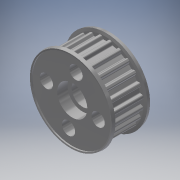
# Autodesk Inventor part: Synchrone Riemenscheibe2
Saved by Autodesk Inventor 2018.3 (Build 223284000, 284)
## iProperties
Created: 2018-08-12
Part Number: Synchrone Riemenscheibe2
Material: Steel
Document SubType Name: Modeling
Designer: JochenAlt
Density: 1 g/cm^3
Appearance: Steel
CustomPartVersion: 1
Author: JochenAlt
Autodesk Inventor part; units mm, degrees
ref_plane "YZ Plane" through (0, 0, 0) normal (1, 0, 0) x (0, 1, 0)
ref_plane "XZ Plane" through (0, 0, 0) normal (0, 1, 0) x (-1, 0, 0)
ref_plane "XY Plane" through (0, 0, 0) normal (0, 0, 1) x (1, 0, 0)
sketch "Riemenscheibenskizze" plane through (0, 0, 0) normal (0, 0, 1) x (1, 0, 0)
  circle A0 centre (0, 0) radius 9.5493 construction
  circle A1 centre (0, 0) radius 9.2493
  circle A2 centre (0, 0) radius 8.4993
  line L0 (-0.8562, 9.2096) -> (-0.525, 8.4993)
  line L1 (-0.525, 8.4993) -> (0.525, 8.4993)
  line L2 (0.525, 8.4993) -> (0.8562, 9.2096)
  line L3 (0, 0) -> (0, 9.2493) construction
  point P0 (0, 8.4993)
  dimension "d0" = 19.0986
  dimension "d1" = 0.3
  dimension "d2" = 0.75
  dimension "d3" = 50
  dimension "d4" = 1.05
  constraints: 8 end point, 3 coincident, 3 point on circle, 2 centre point, 1 horizontal, 1 midpoint, 1 point on line, 1 vertical, 1 vertical alignment, 3 other
  measures "d0" diameter of A0
  measures "d1" radial gap between concentric circles of A0 A1
  measures "d3" angle of L2 L0
  measures "d4" distance of L0.end L1.end
extrude "Grundkörper" add sketch "Riemenscheibenskizze" along normal mid plane 7.5 contours A2 | A1 L0 L1 L2 | L2 L1 L0 A1
extrude "Zahn" cut sketch "Riemenscheibenskizze" along normal through all both and the other way through all contours L2 L1 L0 A1 picked at (0, 8.9964)
fillet "Fillet" radius 0.2 2 edges at (0.525, 8.4993, 0) (-0.525, 8.4993, 0)
fillet "Fillet" radius 0.3 4 edges at (-0.8562, 9.2096, 1.875) (-0.8562, 9.2096, -1.875) (0.8562, 9.2096, 1.875) (0.8562, 9.2096, -1.875)
pattern_circular "Zähne" count 24 over 360 about axis through (0, 0, -10) along (0, 0, 1) of "Zahn", "Fillet"
pulley flange "Flansch links" diameter 18.4986 height 0.8 thickness 0.8 bend angle 10 centre (0, 0, -3.75) toward (0, 0, -1)
pulley flange "Flansch rechts" diameter 18.4986 height 0.8 thickness 0.8 bend angle 10 centre (0, 0, 3.75) toward (0, 0, 1)
sketch "Skizze3" plane through (0, 0, -4.55) normal (0, 0, -1) x (-1, 0, 0)
  circle A0 centre (0, 0) radius 6.35 construction
  line L0 (-14.069, 0) -> (14.069, 0) construction
  circle A1 centre (-0.9037, 6.2854) radius 1.6
  circle A2 centre (0, 0) radius 10.0493 projected
  circle A3 centre (0, 0) radius 9.6
  line L1 (0, -14.069) -> (0, 14.069) construction
  line L2 (14.069, 0) -> (-14.069, 0) construction
  line L3 (0, 0) -> (-0.9037, 6.2854) construction
  circle A4 centre (0, 0) radius 3.65
  circle A5 centre (0, 0) radius 2.65
  circle A6 centre (-0.9037, 6.2854) radius 2.5
  circle A7 centre (-6.2854, -0.9037) radius 1.6
  circle A8 centre (-6.2854, -0.9037) radius 2.5
  circle A9 centre (0.9037, -6.2854) radius 1.6
  circle A10 centre (0.9037, -6.2854) radius 2.5
  circle A11 centre (6.2854, 0.9037) radius 1.6
  circle A12 centre (6.2854, 0.9037) radius 2.5
  dimension "d24" = 6.35
  dimension "d25" = 3.2
  dimension "d30" = 19.2
  dimension "d35" = 8.182
  dimension "d36" = 7.3
  dimension "d38" = 1
  dimension "d43" = 5
  dimension "d46" = 360
  constraints: 12 centre point, 5 coincident, 2 end point, 2 point on circle, 1 point on line, 17 other
  measures "d24" radius of A0
  measures "d25" diameter of A1
  measures "d30" diameter of A3
  measures "d35" angle of L1 L3
  measures "d36" diameter of A4
  measures "d38" radial gap between concentric circles of A4 A5
  measures "d43" diameter of A6
extrude "Extrusion4" cut sketch "Skizze3" against normal through all contours A1 | A7 | A9 | A11
extrude "Extrusion5" cut sketch "Skizze3" along normal blind 0.25 and the other way blind 0.5 from surface at -9.1 contours A1 | A3 | A4 | A5 | A6 | A7 | A8 | A9 | A10 | A11 | A12
extrude "Extrusion6" cut sketch "Skizze3" against normal blind 2.5 contours A4 | A5
extrude "Extrusion9" cut sketch "Skizze3" along normal blind 2.5 from surface at -8.85 contours A4 | A5
extrude "Extrusion10" cut sketch "Skizze3" against normal through all contours A5
equation "\"d1\" = da_a"
equation "\"d2\" = da_hg"
equation "\"d3\" = 2 * da_fi"
equation "\"d4\" = da_bw"
equation "\"d5\" = da_bf"
equation "\"d7\" = da_bf"
equation "\"d9\" = da_rb"
equation "\"d10\" = da_rt"
equation "\"da_pb\" = 2.5"
equation "\"da_fi\" = 25deg"
equation "\"da_hg\" = 0.75"
equation "\"da_bw\" = 1.05"
equation "\"da_rb\" = 0.2"
equation "\"da_rt\" = 0.3"
equation "\"da_a\" = 0.3"
equation "\"da_bf\" = 7.5"
equation "\"da_wf\" = 0.8"
equation "\"da_hf\" = 0.8"
body "Solid1"
